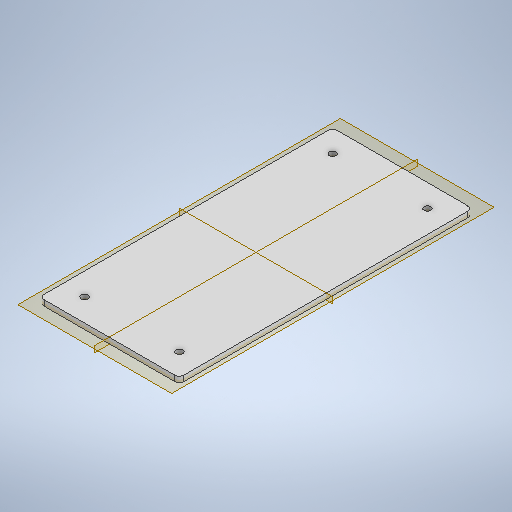
# Autodesk Inventor part: Resistencia_Tapa
Saved by Autodesk Inventor 2026 (Build 300175050, 175E)
## iProperties
Created: 2025-05-26
Part Number: Resistencia_Tapa
Material: Genérico
Document SubType Name: Modeling
Designer: alex
Density: 1 g/cm^3
Appearance: Valor por defecto
Author: alex
Autodesk Inventor part; units mm, degrees
sketch "Tapa" plane through (0, 0, 0) normal (0, 1, 0) x (-1, 0, 0)
  line L0 (29, -65) -> (-29, -65)
  line L1 (-31, -63) -> (-31, 63)
  line L2 (-29, 65) -> (29, 65)
  line L3 (31, 63) -> (31, -63)
  line L4 (0, -91.5799) -> (0, 91.5799) projected
  line L5 (-43.9799, 0) -> (43.9799, 0) projected
  circle A0 centre (21, -55) radius 1.5
  circle A1 centre (-21, -55) radius 1.5
  circle A2 centre (21, 55) radius 1.5
  circle A3 centre (-21, 55) radius 1.5
  arc A4 (29, -65) -> (31, -63) centre (29, -63) ccw
  arc A5 (-31, -63) -> (-29, -65) centre (-29, -63) ccw
  arc A6 (31, 63) -> (29, 65) centre (29, 63) ccw
  arc A7 (-29, 65) -> (-31, 63) centre (-29, 63) ccw
  point P0 (0, 0)
  dimension "d0" = 31
  dimension "d1" = 31
  dimension "d3" = 65
  dimension "d4" = 65
  dimension "d5" = 10
  dimension "d6" = 10
  dimension "d7" = 10
  dimension "d8" = 10
  dimension "d9" = 10
  dimension "d10" = 10
  dimension "d11" = 10
  dimension "d12" = 10
  dimension "d13" = 3
  dimension "d14" = 3
  dimension "d15" = 3
  dimension "d16" = 3
  dimension "d17" = 2
  constraints: 8 centre point, 8 end point, 8 point on circle, 8 tangent, 4 coincident, 3 equal radius, 2 parallel, 1 horizontal, 1 perpendicular
  measures "d0" distance between parallel lines of L1 L4
  measures "d1" distance between parallel lines of L3 L4
  measures "d3" distance between parallel lines of L0 L5
  measures "d4" distance between parallel lines of L5 L2
  measures "d5" distance from line of L1 point (-21, -55)
  measures "d6" distance from line of L0 point (-21, -55)
  measures "d7" distance from line of L0 point (21, -55)
  measures "d8" distance from line of L3 point (21, -55)
  measures "d9" distance from line of L2 point (-21, 55)
  measures "d10" distance from line of L1 point (-21, 55)
  measures "d11" distance from line of L3 point (21, 55)
  measures "d12" distance from line of L2 point (21, 55)
  measures "d13" diameter of A0
  measures "d14" diameter of A1
  measures "d15" diameter of A2
  measures "d16" diameter of A3
  measures "d17" radius of A4
extrude "Extrusión1" add sketch "Tapa" along normal mid plane 2.5
equation "\"d6\" = d5"
equation "\"d7\" = d5"
equation "\"d8\" = d5"
equation "\"d9\" = d5"
equation "\"d10\" = d5"
equation "\"d11\" = d5"
equation "\"d12\" = d5"
equation "\"d14\" = d13"
equation "\"d15\" = d13"
equation "\"d16\" = d13"
